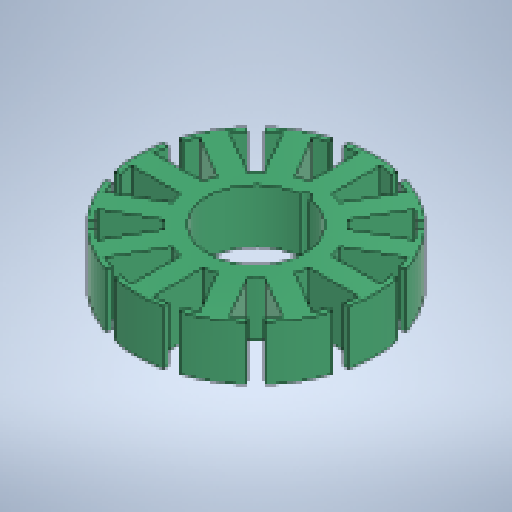
# Autodesk Inventor part: STATOR
Saved by Autodesk Inventor 2023.2 (Build 272271000, 271)
## iProperties
Created: 2024-01-31
Part Number: STATOR
Material: Stainless Steel
Document SubType Name: Modeling
Designer: Nathan Cai
Density: 8 g/cm^3
Appearance: Smooth - Dark Sea Green
Author: Nathan Cai
Autodesk Inventor part; units mm, degrees
ref_plane "YZ Plane" through (0, 0, 0) normal (1, 0, 0) x (0, 1, 0)
ref_plane "XZ Plane" through (0, 0, 0) normal (0, 1, 0) x (-1, 0, 0)
ref_plane "XY Plane" through (0, 0, 0) normal (0, 0, 1) x (1, 0, 0)
sketch "Sketch1" plane through (0, 0, 0) normal (0, 1, 0) x (-1, 0, 0)
  circle A0 centre (0, 0) radius 4.5
  circle A1 centre (0, 0) radius 11
  circle A2 centre (0, 0) radius 6
  circle A3 centre (0, 0) radius 10.5
  line L0 (0, 0) -> (11, 0) construction
  line L1 (5.9161, 1) -> (10.9545, 1)
  line L2 (10.9545, 1) -> (10.9545, -1) construction
  line L3 (10.9545, -1) -> (5.9161, -1)
  line L4 (5.9161, -1) -> (5.9161, 1) construction
  line L5 (5.9161, 1) -> (10.9545, -1) construction
  line L6 (10.9545, 1) -> (5.9161, -1) construction
  line L7 (9.9868, 4.6112) -> (5.6235, 2.092)
  line L8 (4.6235, 3.8241) -> (8.9868, 6.3433)
  line L9 (6.3433, 8.9868) -> (3.8241, 4.6235)
  line L10 (2.092, 5.6235) -> (4.6112, 9.9868)
  line L11 (1, 10.9545) -> (1, 5.9161)
  line L12 (-1, 5.9161) -> (-1, 10.9545)
  line L13 (-4.6112, 9.9868) -> (-2.092, 5.6235)
  line L14 (-3.8241, 4.6235) -> (-6.3433, 8.9868)
  line L15 (-8.9868, 6.3433) -> (-4.6235, 3.8241)
  line L16 (-5.6235, 2.092) -> (-9.9868, 4.6112)
  line L17 (-10.9545, 1) -> (-5.9161, 1)
  line L18 (-5.9161, -1) -> (-10.9545, -1)
  line L19 (-9.9868, -4.6112) -> (-5.6235, -2.092)
  line L20 (-4.6235, -3.8241) -> (-8.9868, -6.3433)
  line L21 (-6.3433, -8.9868) -> (-3.8241, -4.6235)
  line L22 (-2.092, -5.6235) -> (-4.6112, -9.9868)
  line L23 (-1, -10.9545) -> (-1, -5.9161)
  line L24 (1, -5.9161) -> (1, -10.9545)
  line L25 (4.6112, -9.9868) -> (2.092, -5.6235)
  line L26 (3.8241, -4.6235) -> (6.3433, -8.9868)
  line L27 (8.9868, -6.3433) -> (4.6235, -3.8241)
  line L28 (5.6235, -2.092) -> (9.9868, -4.6112)
  line L29 (10.2705, -2.1831) -> (10.7596, -2.287)
  line L30 (10.2705, 2.1831) -> (10.7596, 2.287)
  line L31 (9.9861, 3.2447) -> (10.4616, 3.3992)
  line L32 (7.803, 7.0259) -> (8.1746, 7.3604)
  line L33 (7.0259, 7.803) -> (7.3604, 8.1746)
  line L34 (3.2447, 9.9861) -> (3.3992, 10.4616)
  line L35 (2.1831, 10.2705) -> (2.287, 10.7596)
  line L36 (-2.1831, 10.2705) -> (-2.287, 10.7596)
  line L37 (-3.2447, 9.9861) -> (-3.3992, 10.4616)
  line L38 (-7.0259, 7.803) -> (-7.3604, 8.1746)
  line L39 (-7.803, 7.0259) -> (-8.1746, 7.3604)
  line L40 (-9.9861, 3.2447) -> (-10.4616, 3.3992)
  line L41 (-10.2705, 2.1831) -> (-10.7596, 2.287)
  line L42 (-10.2705, -2.1831) -> (-10.7596, -2.287)
  line L43 (-9.9861, -3.2447) -> (-10.4616, -3.3992)
  line L44 (-7.803, -7.0259) -> (-8.1746, -7.3604)
  line L45 (-7.0259, -7.803) -> (-7.3604, -8.1746)
  line L46 (-3.2447, -9.9861) -> (-3.3992, -10.4616)
  line L47 (-2.1831, -10.2705) -> (-2.287, -10.7596)
  line L48 (2.1831, -10.2705) -> (2.287, -10.7596)
  line L49 (3.2447, -9.9861) -> (3.3992, -10.4616)
  line L50 (7.0259, -7.803) -> (7.3604, -8.1746)
  line L51 (7.803, -7.0259) -> (8.1746, -7.3604)
  line L52 (9.9861, -3.2447) -> (10.4616, -3.3992)
  point P0 (8.4353, 0)
  point P1 (8.4353, 1)
  point P2 (6.8052, 5.0837)
  point P3 (3.3516, 7.8052)
  point P4 (-1, 8.4353)
  point P5 (-5.0837, 6.8052)
  point P6 (-7.8052, 3.3516)
  point P7 (-8.4353, -1)
  point P8 (-6.8052, -5.0837)
  point P9 (-3.3516, -7.8052)
  point P10 (1, -8.4353)
  point P11 (5.0837, -6.8052)
  point P12 (7.8052, -3.3516)
  point P13 (9.9861, -3.2447)
  point P14 (9.5519, -4.3601)
  point P15 (10.4523, -1)
  point P16 (10.2705, 2.1831)
  point P17 (10.4523, 1)
  point P18 (9.5519, 4.3601)
  point P19 (9.9861, 3.2447)
  point P20 (7.803, 7.0259)
  point P21 (8.5519, 6.0922)
  point P22 (6.0922, 8.5519)
  point P23 (7.0259, 7.803)
  point P24 (3.2447, 9.9861)
  point P25 (4.3601, 9.5519)
  point P26 (1, 10.4523)
  point P27 (2.1831, 10.2705)
  point P28 (-1, 10.4523)
  point P29 (-4.3601, 9.5519)
  point P30 (-6.0922, 8.5519)
  point P31 (-8.5519, 6.0922)
  point P32 (-7.803, 7.0259)
  point P33 (-9.9861, 3.2447)
  point P34 (-9.5519, 4.3601)
  point P35 (-10.4523, 1)
  point P36 (-10.2705, 2.1831)
  point P37 (-10.2705, -2.1831)
  point P38 (-10.4523, -1)
  point P39 (-9.5519, -4.3601)
  point P40 (-9.9861, -3.2447)
  point P41 (-7.803, -7.0259)
  point P42 (-8.5519, -6.0922)
  point P43 (-6.0922, -8.5519)
  point P44 (-7.0259, -7.803)
  point P45 (-3.2447, -9.9861)
  point P46 (-4.3601, -9.5519)
  point P47 (-1, -10.4523)
  point P48 (-2.1831, -10.2705)
  point P49 (2.1831, -10.2705)
  point P50 (1, -10.4523)
  point P51 (4.3601, -9.5519)
  point P52 (3.2447, -9.9861)
  point P53 (6.0922, -8.5519)
  point P54 (8.5519, -6.0922)
  point P55 (7.803, -7.0259)
  dimension "d1" = 22
  dimension "d2" = 12
  dimension "d3" = 0.5
  dimension "d0" = 9
  dimension "d4" = 2
  dimension "d7" = 360
  dimension "d9" = 12
  dimension "d12" = 360
  constraints: 106 end point, 13 point on line, 3 coincident, 3 midpoint, 2 horizontal, 2 parallel, 2 symmetric about line, 1 centre point, 1 perpendicular, 181 other
  measures "d0" diameter of A0
  measures "d4" distance from line of point (8.435, 1) L3
  measures "d9" angle of L29 L0
extrude "Extrusion1" add sketch "Sketch1" along normal blind 5 contours A1 L3 A3 L1 | L1 A3 L30 A1 | A1 L29 A3 L3 | A3 L3 A2 L1 | L31 A3 L7 A1 | A2 | A1 L28 A3 L52 | L7 A3 L8 A1 | A2 L8 A3 L7 | A1 L27 A3 L28 | L28 A3 L27 A2 | L8 A3 L32 A1 | A1 L51 A3 L27 | A2 L10 A3 L9 | L26 A3 L25 A2 | L33 A3 L9 A1 | A3 L10 A1 L9 | A1 L26 A3 L50 | L26 A1 L25 A3 | A2 L12 A3 L11 | A3 L34 A1 L10 | L24 A3 L23 A2 | L25 A1 L49 A3 | L11 A1 L35 A3 | A3 L12 A1 L11 | L24 A1 L23 A3 | A3 L48 A1 L24 | A2 L14 A3 L13 | A3 L36 A1 L12 | L22 A3 L21 A2 | L23 A1 L47 A3 | L13 A1 L37 A3 | A3 L14 A1 L13 | L22 A1 L21 A3 | A3 L46 A1 L22 | A2 L16 A3 L15 | A3 L38 A1 L14 | L20 A3 L19 A2 | L21 A1 L45 A3 | L15 A1 L39 A3 | A3 L16 A1 L15 | L20 A1 L19 A3 | A3 L44 A1 L20 | A2 L18 A3 L17 | A3 L40 A1 L16 | L19 A1 L43 A3 | L17 A1 L41 A3 | A3 L18 A1 L17 | A3 L42 A1 L18
sketch "Sketch2" plane through (0, 5, 0) normal (0, 1, 0) x (1, 0, 0)
  circle A0 centre (0, 0) radius 4.5 projected
  circle A1 centre (0, 4.5) radius 0.5
  line L0 (0, 0) -> (0, 4.5) construction
  dimension "d16" = 1
  constraints: 2 end point, 1 centre point, 1 vertical, 1 vertical alignment, 1 other
  measures "d16" diameter of A1
extrude "Extrusion2" cut sketch "Sketch2" against normal through all contours A1 A0 | A0 A1 picked at (0.0194, 4.3324) picked at (0.0158, 4.6639)
body "Solid1"
